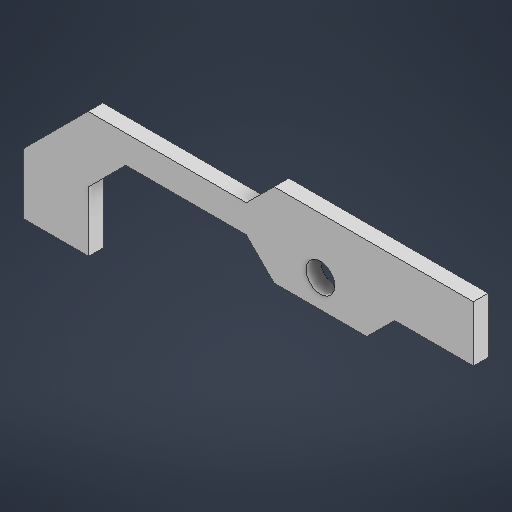
# Autodesk Inventor part: qreMiniBoard2
Saved by Autodesk Inventor 2025 (Build 290162000, 162)
## iProperties
Created: 2025-03-18
Part Number: qreMiniBoard2
Material: Všeobecné
Document SubType Name: Modeling
Designer: Simak
Density: 1 g/cm^3
Appearance: Výchozí
Author: Simak
Autodesk Inventor part; units mm, degrees
ref_plane "YZ Plane" through (0, 0, 0) normal (1, 0, 0) x (0, 1, 0)
ref_plane "XZ Plane" through (0, 0, 0) normal (0, 1, 0) x (-1, 0, 0)
ref_plane "XY Plane" through (0, 0, 0) normal (0, 0, 1) x (1, 0, 0)
sketch "Náčrt1" plane through (0, 0, 0) normal (0, 0, 1) x (1, 0, 0)
  line L0 (0, 3) -> (-21.5, 3)
  line L1 (-21.5, 3) -> (-24.5, 0)
  line L2 (-24.5, 0) -> (-41.5711, 0)
  line L3 (-41.5711, 0) -> (-48.5, -6.9289)
  line L4 (-48.5, -6.9289) -> (-48.5, -13.5)
  line L5 (-48.5, -13.5) -> (-41.5, -13.5)
  line L6 (-41.5, -13.5) -> (-41.5, -7)
  line L7 (-41.5, -7) -> (-37.5, -3)
  line L8 (-37.5, -3) -> (-24.5, -3)
  line L9 (-24.5, -3) -> (-21.5, -6)
  line L10 (-21.5, -6) -> (-11.5, -6)
  line L11 (-11.5, -6) -> (-8.5, -3)
  line L12 (-8.5, -3) -> (0, -3)
  circle A0 centre (-16.5, -3) radius 1.55
  line L13 (-47.5, -13.5) -> (-47.5, -5.9289) construction
  line L14 (0, 3) -> (0, -3)
  point P0 (0, 0)
  point P1 (-16.5, -6)
  point P2 (0, 0)
  dimension "d47" = 3
  dimension "d49" = 45
  dimension "d51" = 3
  dimension "d52" = 48.5
  dimension "d53" = 4
  dimension "d54" = 10.5
  dimension "d55" = 5
  dimension "d56" = 7
  dimension "d57" = 1
  dimension "d58" = 10
  dimension "d59" = 16.5
  dimension "d60" = 3
  dimension "d62" = 3.1
  dimension "d64" = 21.5
  constraints: 30 end point, 7 parallel, 5 perpendicular, 3 vertical alignment, 2 midpoint, 2 point on line, 1 centre point, 1 coincident, 1 collinear, 1 horizontal, 1 horizontal alignment, 1 vertical
  measures "d47" distance between parallel lines of L8 L2
  measures "d49" angle of L1 L2
  measures "d51" distance between parallel lines of L2 L0
  measures "d52" distance from line of L12.end L4
  measures "d53" horizontal distance of L6.end L7.end
  measures "d54" distance between parallel lines of L5 L8
  measures "d55" distance between parallel lines of L3 L7
  measures "d56" distance of L4.end L5.end
  measures "d57" distance between parallel lines of L4 L13
  measures "d58" distance of L9.end L10.end
  measures "d59" horizontal distance of L0.start A0.centre
  measures "d60" distance between parallel lines of L12 L10
  measures "d62" diameter of A0
  measures "d64" distance of L0.start L0.end
extrude "Vysunutí1" add sketch "Náčrt1" along normal blind 1.6
